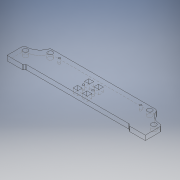
# Autodesk Inventor part: A8-0008
Saved by Autodesk Inventor 2016 SP2 (Build 200236200, 236)
## iProperties
Created: 2017-04-22
Part Number: A8-0008
Material: Generic
Document SubType Name: Modeling
Designer: EV
Density: 1 g/cm^3
Appearance: Default
Author: EV
Autodesk Inventor part; units mm, degrees
ref_plane "YZ Plane" through (0, 0, 0) normal (1, 0, 0) x (0, 1, 0)
ref_plane "XY Plane" through (0, 0, 0) normal (0, 0, 1) x (1, 0, 0)
sketch "Sketch1" plane through (0, 0, 0) normal (0, 1, 0) x (-1, 0, 0)
  line L0 (-117.5, 47) -> (-117.5, 0)
  line L1 (-117.5, 0) -> (117.5, 0)
  line L2 (117.5, 0) -> (117.5, 47)
  line L3 (90.5, 47) -> (87.5, 44)
  line L4 (87.5, 44) -> (-87.5, 44)
  line L5 (-87.5, 44) -> (-90.5, 47)
  line L6 (117.5, 47) -> (90.5, 47)
  line L7 (-90.5, 47) -> (-117.5, 47)
  arc A0 (113.5, 18) -> (117.5, 22) centre (113.5, 22) ccw
  arc A1 (113.5, 18) -> (91, 0) centre (113.5, -5.0625) ccw
  line L8 (113.5, 22) -> (113.5, 18) construction
  arc A2 (-117.5, 22) -> (-113.5, 18) centre (-113.5, 22) ccw
  arc A3 (-91, 0) -> (-113.5, 18) centre (-113.5, -5.0625) ccw
  line L9 (-113.5, 22) -> (-113.5, 18) construction
  line L10 (0, 44) -> (0, 0) construction
  line L11 (13.5, 11.8) -> (5.3, 11.8)
  line L12 (5.3, 11.8) -> (5.3, 19.3)
  line L13 (5.3, 19.3) -> (13.5, 19.3)
  line L14 (13.5, 19.3) -> (13.5, 11.8)
  line L15 (13.5, 31.3) -> (5.3, 31.3)
  line L16 (5.3, 31.3) -> (5.3, 38.8)
  line L17 (5.3, 38.8) -> (13.5, 38.8)
  line L18 (13.5, 38.8) -> (13.5, 31.3)
  line L19 (-2.7, 11.8) -> (-10.9, 11.8)
  line L20 (-10.9, 11.8) -> (-10.9, 19.3)
  line L21 (-10.9, 19.3) -> (-2.7, 19.3)
  line L22 (-2.7, 19.3) -> (-2.7, 11.8)
  line L23 (-2.7, 31.3) -> (-10.9, 31.3)
  line L24 (-10.9, 31.3) -> (-10.9, 38.8)
  line L25 (-10.9, 38.8) -> (-2.7, 38.8)
  line L26 (-2.7, 38.8) -> (-2.7, 31.3)
  dimension "d1" = 235
  dimension "d2" = 3
  dimension "d3" = 45
  dimension "d4" = 27
  dimension "d5" = 47
  dimension "d6" = 4
  dimension "d7" = 29
  dimension "d8" = 23.0625
  dimension "d9" = 182
  dimension "d10" = 8.2
  dimension "d11" = 7.5
  dimension "d12" = 12
  dimension "d14" = 8
  dimension "d15" = 11.8
  dimension "d16" = 104
  dimension "d17" = 106.6
  constraints: 54 end point, 12 parallel, 11 collinear, 8 point on circle, 7 perpendicular, 6 horizontal, 4 centre point, 4 point on line, 3 vertical, 2 equal radius, 2 midpoint, 2 tangent, 1 coincident, 1 vertical alignment, 2 other
  measures "d1" distance of L2.end L0.start
  measures "d2" distance between parallel lines of L7 L4
  measures "d3" angle of L6 L3
  measures "d4" distance of L2.end L3.start
  measures "d5" distance between parallel lines of L1 L6
  measures "d6" radius of A0
  measures "d7" distance from line of L6 L8.end
  measures "d8" radius of A1
  measures "d9" distance of A3.start A1.end
  measures "d10" distance of L16.end L17.end
  measures "d11" distance of L17.end L15.start
  measures "d12" distance between parallel lines of L13 L15
  measures "d14" distance between parallel lines of L16 L26
  measures "d15" distance between parallel lines of L1 L11
  measures "d16" distance between parallel lines of L2 L18
  measures "d17" distance between parallel lines of L0 L24
extrude "Extrusion1" add sketch "Sketch1" along normal blind 8 contours L7 L5 L4 L3 L6 L2 A0 A1 L1 A3 A2 L0
fillet "Fillet1" radius 4 2 edges at (-91, 4, 0) (91, 4, 0)
fillet "Fillet2" radius 2 4 edges at (-90.5, 4, 47) (-87.5, 4, 44) (87.5, 4, 44) (90.5, 4, 47)
sketch "Sketch2" plane through (0, 8, 0) normal (0, 1, 0) x (1, 0, 0)
  arc A0 (89.9142, -46.4142) -> (91.3284, -47) centre (91.3284, -45) ccw construction
  line L0 (91.3284, -47) -> (117.5, -47) construction
  line L1 (117.5, -47) -> (117.5, -22) construction
  arc A1 (117.5, -22) -> (113.5, -18) centre (113.5, -22) ccw construction
  arc A2 (91.7691, -2.6605) -> (113.5, -18) centre (113.5, 5.0625) ccw construction
  arc A3 (91.7691, -2.6605) -> (88, 0) centre (88, -4) ccw construction
  line L2 (88, 0) -> (-88, 0) construction
  arc A4 (-88, 0) -> (-91.7691, -2.6605) centre (-88, -4) ccw construction
  arc A5 (-113.5, -18) -> (-91.7691, -2.6605) centre (-113.5, 5.0625) ccw construction
  arc A6 (-113.5, -18) -> (-117.5, -22) centre (-113.5, -22) ccw construction
  line L3 (-117.5, -22) -> (-117.5, -47) construction
  line L4 (-117.5, -47) -> (-91.3284, -47) construction
  arc A7 (-91.3284, -47) -> (-89.9142, -46.4142) centre (-91.3284, -45) ccw construction
  line L5 (-89.9142, -46.4142) -> (-88.0858, -44.5858) construction
  arc A8 (-86.6716, -44) -> (-88.0858, -44.5858) centre (-86.6716, -46) ccw construction
  line L6 (-86.6716, -44) -> (86.6716, -44) construction
  arc A9 (88.0858, -44.5858) -> (86.6716, -44) centre (86.6716, -46) ccw construction
  line L7 (88.0858, -44.5858) -> (89.9142, -46.4142) construction
  line L8 (10.9, -31.3) -> (10.9, -38.8) construction
  line L9 (10.9, -38.8) -> (2.7, -38.8) construction
  line L10 (2.7, -38.8) -> (2.7, -31.3) construction
  line L11 (2.7, -31.3) -> (10.9, -31.3) construction
  line L12 (10.9, -11.8) -> (10.9, -19.3) construction
  line L13 (10.9, -19.3) -> (2.7, -19.3) construction
  line L14 (2.7, -19.3) -> (2.7, -11.8) construction
  line L15 (2.7, -11.8) -> (10.9, -11.8) construction
  line L16 (-5.3, -31.3) -> (-5.3, -38.8) construction
  line L17 (-5.3, -38.8) -> (-13.5, -38.8) construction
  line L18 (-13.5, -38.8) -> (-13.5, -31.3) construction
  line L19 (-13.5, -31.3) -> (-5.3, -31.3) construction
  line L20 (-5.3, -11.8) -> (-5.3, -19.3) construction
  line L21 (-5.3, -19.3) -> (-13.5, -19.3) construction
  line L22 (-13.5, -19.3) -> (-13.5, -11.8) construction
  line L23 (-13.5, -11.8) -> (-5.3, -11.8) construction
  line L24 (-13.5, -31.3) -> (-5.3, -31.3) construction
  line L25 (-9.4, -31.3) -> (-9.4, -19.3) construction
  line L26 (-5.3, -19.3) -> (-13.5, -19.3) construction
  line L27 (10.9, -31.3) -> (2.7, -31.3) construction
  line L28 (6.8, -31.3) -> (6.8, -19.3) construction
  point P0 (0, 0)
  point P1 (-9.4, -25.3)
  point P2 (6.8, -25.3)
  point P3 (-109, -24)
  point P4 (-85.5, -6.5)
  point P5 (-69, -6.5)
  point P6 (85.5, -6.5)
  point P7 (69, -6.5)
  point P8 (109, -24)
  dimension "d22" = 23
  dimension "d23" = 8.5
  dimension "d24" = 6.5
  dimension "d25" = 32
  dimension "d26" = 48.5
  dimension "d27" = 8.5
  dimension "d29" = 48.5
  dimension "d30" = 32
  constraints: 6 midpoint, 4 end point, 4 horizontal alignment
  measures "d22" distance from line of point (-109, -24) L4
  measures "d23" distance from line of L3 point (-109, -24)
  measures "d24" distance from line of L2 point (-85.5, -6.5)
  measures "d25" distance from line of L3 point (-85.5, -6.5)
  measures "d26" distance from line of L3 point (-69, -6.5)
  measures "d27" distance from line of point (109, -24) L1
  measures "d29" distance from line of L1 point (69, -6.5)
  measures "d30" distance from line of L1 point (85.5, -6.5)
hole "Hole1" at (-9.4, 8, 25.3) at (6.8, 8, 25.3) at (-69, 8, 6.5) at (69, 8, 6.5) direction (0, -1, 0) diameter 3.5 end through all
hole "Hole2" at (-109, 8, 24) at (-85.5, 8, 6.5) at (85.5, 8, 6.5) at (109, 8, 24) direction (0, -1, 0) diameter 8.2 end through all
ref_plane "Work Plane1" through (-117.5, 0, 47) normal (0, 0, 1) x (1, 0, 0)
equation "\"d27\" = d23"
equation "\"d29\" = d26"
equation "\"d30\" = d25"
body "Solid1"
